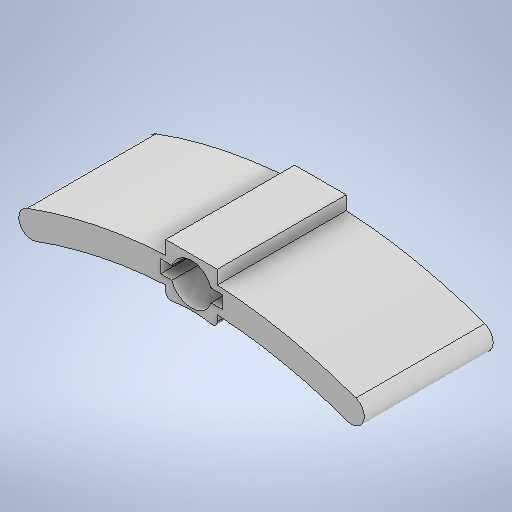
# Autodesk Inventor part: sorter
Saved by Autodesk Inventor 2025.4 (Build 294407000, 407)
## iProperties
Created: 2026-03-10
Part Number: sorter
Material: Generic
Document SubType Name: Modeling
Designer: Amir
Density: 1 g/cm^3
Appearance: Default
Author: Amir
## iProperties of the stored document sorter_3DPrint.ipt
Created: 2026-03-11
Part Number: sorter_3DPrint
Material: Generic
Document SubType Name: Modeling
Designer: Amir
Density: 1 g/cm^3
Appearance: Default
Author: Amir
Autodesk Inventor part; units mm, degrees
ref_plane "YZ Plane" through (0, 0, 0) normal (1, 0, 0) x (0, 1, 0)
ref_plane "XZ Plane" through (0, 0, 0) normal (0, 1, 0) x (-1, 0, 0)
ref_plane "XY Plane" through (0, 0, 0) normal (0, 0, 1) x (1, 0, 0)
sketch "Sketch1" plane through (0, 0, 0) normal (0, 0, 1) x (1, 0, 0)
  arc A0 (31, 0) -> (-31, 0) centre (0, -84.0628) ccw construction
  arc A1 (31.865, 2.3456) -> (-31.865, 2.3456) centre (0, -84.0628) ccw
  arc A2 (30.135, -2.3456) -> (-30.135, -2.3456) centre (0, -84.0628) ccw
  arc A3 (30.135, -2.3456) -> (31.865, 2.3456) centre (31, 0) ccw
  arc A4 (-31.865, 2.3456) -> (-30.135, -2.3456) centre (-31, 0) ccw
  line L0 (5, 0.5338) -> (5, 10.5338)
  line L1 (5, 10.5338) -> (-5, 10.5338)
  line L2 (-5, 10.5338) -> (-5, 0.5338)
  line L3 (-5, 0.5338) -> (5, 10.5338) construction
  line L4 (5, 0.5338) -> (-5, 10.5338) construction
  circle A5 centre (0, 5.5338) radius 4
  line L5 (-6, 4.2838) -> (6, 4.2838)
  line L6 (6, 4.2838) -> (6, 6.7838)
  line L7 (6, 6.7838) -> (-6, 6.7838)
  line L8 (-6, 6.7838) -> (-6, 4.2838)
  arc A6 (5, 0.5338) -> (-5, 0.5338) centre (0, -20.4862) ccw
  point P0 (0, 0)
  point P1 (3.7997, 4.2838)
  point P2 (-3.7997, 4.2838)
  point P3 (-3.7997, 6.7838)
  point P4 (3.7997, 6.7838)
  point P5 (5, 2.8902)
  point P6 (5, 7.898)
  point P7 (-5, 7.898)
  point P8 (-5, 2.8902)
  point P9 (3.0781, 2.9794)
  point P10 (-3.0781, 2.9794)
  dimension "d0" = 62
  dimension "d1" = 5
  dimension "d2" = 87.0966
  dimension "d3" = 10
  dimension "d4" = 10
  dimension "d5" = 8
  dimension "d6" = 12
  dimension "d7" = 2.5
  dimension "d8" = 1.25
  constraints: 18 end point, 13 point on circle, 7 centre point, 4 tangent, 3 parallel, 2 horizontal, 2 horizontal alignment, 2 midpoint, 1 coincident, 1 perpendicular, 1 vertical, 1 vertical alignment
  measures "d0" distance of A4.centre A3.centre
  measures "d1" diameter of A3
  measures "d2" radius of A2
  measures "d3" distance of L1.end L0.end
  measures "d4" distance of L0.end L0.start
  measures "d5" diameter of A5
  measures "d6" distance of L7.end L6.end
  measures "d7" distance of L6.end L5.end
  measures "d8" distance from line of A5.centre L5
extrude "Extrusion1" add sketch "Sketch1" along normal blind 25 contours A3 A2 L0 L5 L6 L7 A1 | L0 L7 A5 A1 | A1 A5 L2 L1 L0 | L0 A6 L2 A2 A5 | A2 A5 L5 L0 | A5 L7 L2 A1 | L2 L7 L8 L5 A2 A4 A1 | A2 L2 L5 A5
fillet "Fillet2" radius 1 1 edges at (5, 0.5338, 12.5)
fillet "Fillet3" radius 1 1 edges at (-5, 0.5338, 12.5)
body "Solid1"
